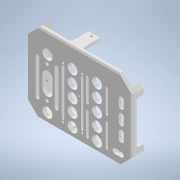
# Autodesk Inventor part: pcb_shell_1
Saved by Autodesk Inventor 2020 (Build 240168000, 168)
## iProperties
Created: 2019-07-14
Part Number: pcb_shell_1
Material: Generic
Document SubType Name: Modeling
Designer: psrob
Density: 1 g/cm^3
Appearance: Default
Author: psrob
Autodesk Inventor part; units mm, degrees
(part 1 of 2)
ref_plane "YZ Plane" through (0, 0, 0) normal (1, 0, 0) x (0, 1, 0)
ref_plane "XZ Plane" through (0, 0, 0) normal (0, 1, 0) x (-1, 0, 0)
ref_plane "XY Plane" through (0, 0, 0) normal (0, 0, 1) x (1, 0, 0)
sketch "Sketch1" plane through (0, 0, 0) normal (0, 0, 1) x (1, 0, 0)
  circle A0 centre (-25.7325, -16.0275) radius 1.27 projected
  circle A1 centre (-25.7325, 9.3725) radius 1.27 projected
  circle A2 centre (-13.0275, 16.3575) radius 0.889 projected
  circle A3 centre (2.2125, 16.3575) radius 0.889 projected
  circle A4 centre (2.2125, -24.2825) radius 0.889 projected
  circle A5 centre (-13.0275, -24.2825) radius 0.889 projected
  circle A6 centre (28.3275, -23.6475) radius 0.65 projected
  circle A7 centre (33.3275, -23.6475) radius 0.65 projected
  circle A8 centre (33.3275, -13.4075) radius 0.65 projected
  circle A9 centre (33.3275, -8.4075) radius 0.65 projected
  circle A10 centre (33.3275, -1.9775) radius 0.65 projected
  circle A11 centre (33.3275, 3.0225) radius 0.65 projected
  circle A12 centre (33.3275, 9.4525) radius 0.65 projected
  circle A13 centre (33.3275, 14.4525) radius 0.65 projected
  circle A14 centre (-33.3425, 10.6425) radius 0.555 projected
  circle A15 centre (-33.3425, 8.1025) radius 0.555 projected
  circle A16 centre (-33.3425, 5.5625) radius 0.555 projected
  circle A17 centre (-33.3425, 3.0225) radius 0.555 projected
  circle A18 centre (-33.3425, 0.4825) radius 0.555 projected
  circle A19 centre (-33.3425, -2.0575) radius 0.555 projected
  circle A20 centre (-33.3425, -4.5975) radius 0.555 projected
  circle A21 centre (-33.3425, -7.1375) radius 0.555 projected
  circle A22 centre (-33.3425, -9.6775) radius 0.555 projected
  circle A23 centre (-33.3425, -12.2175) radius 0.555 projected
  circle A24 centre (-33.3425, -14.7575) radius 0.555 projected
  circle A25 centre (-33.3425, -17.2975) radius 0.555 projected
  circle A26 centre (-18.1125, -17.2975) radius 0.555 projected
  circle A27 centre (-18.1125, -14.7575) radius 0.555 projected
  circle A28 centre (-18.1125, -12.2175) radius 0.555 projected
  circle A29 centre (-18.1125, -9.6775) radius 0.555 projected
  circle A30 centre (-18.1125, -7.1375) radius 0.555 projected
  circle A31 centre (-18.1125, -4.5975) radius 0.555 projected
  circle A32 centre (-18.1125, -2.0575) radius 0.555 projected
  circle A33 centre (-18.1125, 0.4825) radius 0.555 projected
  circle A34 centre (-18.1125, 3.0225) radius 0.555 projected
  circle A35 centre (-18.1125, 5.5625) radius 0.555 projected
  circle A36 centre (-18.1125, 8.1025) radius 0.555 projected
  circle A37 centre (-18.1125, 10.6425) radius 0.555 projected
  circle A38 centre (2.2075, -21.7475) radius 0.4 projected
  circle A39 centre (2.2075, -19.1975) radius 0.4 projected
  circle A40 centre (2.2075, -16.6675) radius 0.4 projected
  circle A41 centre (2.2075, -14.1175) radius 0.4 projected
  circle A42 centre (2.2075, -11.5775) radius 0.4 projected
  circle A43 centre (2.2075, -9.0475) radius 0.4 projected
  circle A44 centre (2.2075, -6.4975) radius 0.4 projected
  circle A45 centre (2.2075, -3.9575) radius 0.4 projected
  circle A46 centre (2.2075, -1.4175) radius 0.4 projected
  circle A47 centre (2.2075, 1.1225) radius 0.4 projected
  circle A48 centre (2.2075, 3.6625) radius 0.4 projected
  circle A49 centre (2.2075, 6.2025) radius 0.4 projected
  circle A50 centre (2.2075, 8.7425) radius 0.4 projected
  circle A51 centre (2.2075, 11.2725) radius 0.4 projected
  circle A52 centre (2.2075, 13.8125) radius 0.4 projected
  circle A53 centre (-13.0225, 13.8125) radius 0.4 projected
  circle A54 centre (-13.0225, 11.2725) radius 0.4 projected
  circle A55 centre (-13.0225, 8.7425) radius 0.4 projected
  circle A56 centre (-13.0225, 6.2025) radius 0.4 projected
  circle A57 centre (-13.0225, 3.6625) radius 0.4 projected
  circle A58 centre (-13.0225, 1.1225) radius 0.4 projected
  circle A59 centre (-13.0225, -1.4175) radius 0.4 projected
  circle A60 centre (-13.0225, -3.9575) radius 0.4 projected
  circle A61 centre (-13.0225, -6.4975) radius 0.4 projected
  circle A62 centre (-13.0225, -9.0475) radius 0.4 projected
  circle A63 centre (-13.0225, -11.5775) radius 0.4 projected
  circle A64 centre (-13.0225, -14.1175) radius 0.4 projected
  circle A65 centre (-13.0225, -16.6675) radius 0.4 projected
  circle A66 centre (-13.0225, -19.1975) radius 0.4 projected
  circle A67 centre (-13.0225, -21.7475) radius 0.4 projected
  circle A68 centre (21.8975, -7.1375) radius 0.35 projected
  circle A69 centre (21.8975, 16.3625) radius 0.35 projected
  circle A70 centre (21.8975, -9.6775) radius 0.3 projected
  circle A71 centre (6.4075, -14.7575) radius 0.3 projected
  circle A72 centre (6.4075, -22.3775) radius 0.3 projected
  circle A73 centre (6.4075, -7.1375) radius 0.3 projected
  circle A74 centre (6.4075, -24.9175) radius 0.3 projected
  circle A75 centre (21.8975, -24.9175) radius 0.3 projected
  circle A76 centre (21.8975, -12.2175) radius 0.3 projected
  circle A77 centre (6.4075, -19.8375) radius 0.3 projected
  circle A78 centre (6.4075, -17.2975) radius 0.3 projected
  circle A79 centre (21.8975, -19.8375) radius 0.3 projected
  circle A80 centre (21.8975, -22.3775) radius 0.3 projected
  circle A81 centre (6.4075, -9.6775) radius 0.3 projected
  circle A82 centre (6.4075, -12.2175) radius 0.3 projected
  circle A83 centre (21.8975, -17.2975) radius 0.3 projected
  circle A84 centre (21.8975, -14.7575) radius 0.3 projected
  circle A85 centre (21.8975, 13.8125) radius 0.3 projected
  circle A86 centre (6.4075, 8.7425) radius 0.3 projected
  circle A87 centre (6.4075, 1.1225) radius 0.3 projected
  circle A88 centre (6.4075, 16.3625) radius 0.3 projected
  circle A89 centre (6.4075, -1.4175) radius 0.3 projected
  circle A90 centre (21.8975, -1.4175) radius 0.3 projected
  circle A91 centre (21.8975, 11.2725) radius 0.3 projected
  circle A92 centre (6.4075, 3.6625) radius 0.3 projected
  circle A93 centre (6.4075, 6.2025) radius 0.3 projected
  circle A94 centre (21.8975, 3.6625) radius 0.3 projected
  circle A95 centre (21.8975, 1.1225) radius 0.3 projected
  circle A96 centre (6.4075, 13.8125) radius 0.3 projected
  circle A97 centre (6.4075, 11.2725) radius 0.3 projected
  circle A98 centre (21.8975, 6.2025) radius 0.3 projected
  circle A99 centre (21.8975, 8.7425) radius 0.3 projected
  circle A100 centre (11.0517, 18.7705) radius 0.175 projected
  circle A101 centre (4.7779, 21.7423) radius 0.175 projected
  circle A102 centre (15.3443, 11.8363) radius 0.175 projected
  circle A103 centre (29.2127, 21.7423) radius 0.175 projected
  circle A104 centre (-2.8167, 21.4121) radius 0.175 projected
  circle A105 centre (-15.0341, 10.8457) radius 0.175 projected
  line L0 (37.1375, -27.4575) -> (-37.1375, -27.4575) projected
  line L1 (37.1375, 27.4575) -> (37.1375, -27.4575) projected
  line L2 (-37.1375, 27.4575) -> (37.1375, 27.4575) projected
  line L3 (-37.1375, -27.4575) -> (-37.1375, 27.4575) projected
  line L4 (-39, 29) -> (39, 29)
  line L5 (39, 29) -> (39, -29)
  line L6 (39, -29) -> (-39, -29)
  line L7 (-39, -29) -> (-39, 29)
  line L8 (-39, 29) -> (39, -29) construction
  line L9 (39, 29) -> (-39, -29) construction
  line L10 (-42, 31.5) -> (42, 31.5)
  line L11 (42, 31.5) -> (42, -31.5)
  line L12 (42, -31.5) -> (-42, -31.5)
  line L13 (-42, -31.5) -> (-42, 31.5)
  line L14 (-42, 31.5) -> (42, -31.5) construction
  line L15 (42, 31.5) -> (-42, -31.5) construction
  point P0 (0, 0)
  dimension "d0" = 78
  dimension "d1" = 58
  dimension "d2" = 84
  dimension "d3" = 63
  constraints: 24 end point, 4 midpoint, 4 parallel, 3 perpendicular, 1 horizontal
  measures "d0" distance of L4.start L4.end
  measures "d1" distance of L4.end L5.end
  measures "d2" distance of L10.start L10.end
  measures "d3" distance of L10.end L11.end
extrude "Extrusion1" add sketch "Sketch1" along normal blind 3 contours A0 | A1 | A2 | A3 | A4 | A5 | A6 | A7 | A8 | A9 | A10 | A11 | A12 | A13 | A14 | A15 | A16 | A17 | A18 | A19 | A20 | A21 | A22 | A23 | A24 | A25 | A26 | A27 | A28 | A29 | A30 | A31 | A32 | A33 | A34 | A35 | A36 | A37 | A38 | A39 | A40 | A41 | A42 | A43 | A44 | A45 | A46 | A47 | A48 | A49 | A50 | A51 | A52 | A53 | A54 | A55 | A56 | A57 | A58 | A59 | A60 | A61 | A62 | A63 | A64 | A65 | A66 | A67 | A68 | A69 | A70 | A71 | A72 | A73 | A74 | A75 | A76 | A77 | A78 | A79 | A80 | A81 | A82 | A83 | A84 | A85 | A86 | A87 | A88 | A89 | A90 | A91 | A92 | A93 | A94 | A95 | A96 | A97 | A98 | A99 | A100 | A101 | A102 | A103 | A104 | A105 | L0 L3 L2 L1 | L4 L5 L6 L7 | L10 L11 L12 L13
sketch "Sketch2" plane through (0, 0, 0) normal (0, 0, -1) x (-1, 0, 0)
  line L0 (42, -31.5) -> (-42, -31.5) projected
  line L1 (42, 31.5) -> (42, -31.5) projected
  line L2 (-42, 31.5) -> (42, 31.5) projected
  line L3 (-42, -31.5) -> (-42, 31.5) projected
  line L4 (39, -29) -> (-39, -29)
  line L5 (-39, -29) -> (-39, 29)
  line L6 (-39, 29) -> (39, 29)
  line L7 (39, 29) -> (39, -29)
  line L8 (39, -29) -> (-39, 29) construction
  line L9 (-39, -29) -> (39, 29) construction
  point P0 (0, 0)
  dimension "d6" = 78
  dimension "d7" = 58
  constraints: 12 end point, 2 midpoint, 2 parallel, 1 horizontal, 1 perpendicular
  measures "d6" distance of L4.start L4.end
  measures "d7" distance of L4.end L5.end
extrude "Extrusion2" add sketch "Sketch2" along normal blind 14
sketch "Sketch3" plane through (0, 0, 3) normal (0, 0, 1) x (1, 0, 0)
  circle A0 centre (-25.7325, -16.0275) radius 1.27 projected
  circle A1 centre (-25.7325, 9.3725) radius 1.27 projected
  circle A2 centre (-13.0275, 16.3575) radius 0.889 projected
  circle A3 centre (2.2125, 16.3575) radius 0.889 projected
  circle A4 centre (2.2125, -24.2825) radius 0.889 projected
  circle A5 centre (-13.0275, -24.2825) radius 0.889 projected
  circle A6 centre (28.3275, -23.6475) radius 0.65 projected
  circle A7 centre (33.3275, -23.6475) radius 0.65 projected
  circle A8 centre (33.3275, -13.4075) radius 0.65 projected
  circle A9 centre (33.3275, -8.4075) radius 0.65 projected
  circle A10 centre (33.3275, -1.9775) radius 0.65 projected
  circle A11 centre (33.3275, 3.0225) radius 0.65 projected
  circle A12 centre (33.3275, 9.4525) radius 0.65 projected
  circle A13 centre (33.3275, 14.4525) radius 0.65 projected
  circle A14 centre (-33.3425, 10.6425) radius 0.555 projected
  circle A15 centre (-33.3425, 8.1025) radius 0.555 projected
  circle A16 centre (-33.3425, 5.5625) radius 0.555 projected
  circle A17 centre (-33.3425, 3.0225) radius 0.555 projected
  circle A18 centre (-33.3425, 0.4825) radius 0.555 projected
  circle A19 centre (-33.3425, -2.0575) radius 0.555 projected
  circle A20 centre (-33.3425, -4.5975) radius 0.555 projected
  circle A21 centre (-33.3425, -7.1375) radius 0.555 projected
  circle A22 centre (-33.3425, -9.6775) radius 0.555 projected
  circle A23 centre (-33.3425, -12.2175) radius 0.555 projected
  circle A24 centre (-33.3425, -14.7575) radius 0.555 projected
  circle A25 centre (-33.3425, -17.2975) radius 0.555 projected
  circle A26 centre (-18.1125, -17.2975) radius 0.555 projected
  circle A27 centre (-18.1125, -14.7575) radius 0.555 projected
  circle A28 centre (-18.1125, -12.2175) radius 0.555 projected
  circle A29 centre (-18.1125, -9.6775) radius 0.555 projected
  circle A30 centre (-18.1125, -7.1375) radius 0.555 projected
  circle A31 centre (-18.1125, -4.5975) radius 0.555 projected
  circle A32 centre (-18.1125, -2.0575) radius 0.555 projected
  circle A33 centre (-18.1125, 0.4825) radius 0.555 projected
  circle A34 centre (-18.1125, 3.0225) radius 0.555 projected
  circle A35 centre (-18.1125, 5.5625) radius 0.555 projected
  circle A36 centre (-18.1125, 8.1025) radius 0.555 projected
  circle A37 centre (-18.1125, 10.6425) radius 0.555 projected
  circle A38 centre (2.2075, -21.7475) radius 0.4 projected
  circle A39 centre (2.2075, -19.1975) radius 0.4 projected
  circle A40 centre (2.2075, -16.6675) radius 0.4 projected
  circle A41 centre (2.2075, -14.1175) radius 0.4 projected
  circle A42 centre (2.2075, -11.5775) radius 0.4 projected
  circle A43 centre (2.2075, -9.0475) radius 0.4 projected
  circle A44 centre (2.2075, -6.4975) radius 0.4 projected
  circle A45 centre (2.2075, -3.9575) radius 0.4 projected
  circle A46 centre (2.2075, -1.4175) radius 0.4 projected
  circle A47 centre (2.2075, 1.1225) radius 0.4 projected
  circle A48 centre (2.2075, 3.6625) radius 0.4 projected
  circle A49 centre (2.2075, 6.2025) radius 0.4 projected
  circle A50 centre (2.2075, 8.7425) radius 0.4 projected
  circle A51 centre (2.2075, 11.2725) radius 0.4 projected
  circle A52 centre (2.2075, 13.8125) radius 0.4 projected
  circle A53 centre (-13.0225, 13.8125) radius 0.4 projected
  circle A54 centre (-13.0225, 11.2725) radius 0.4 projected
  circle A55 centre (-13.0225, 8.7425) radius 0.4 projected
  circle A56 centre (-13.0225, 6.2025) radius 0.4 projected
  circle A57 centre (-13.0225, 3.6625) radius 0.4 projected
  circle A58 centre (-13.0225, 1.1225) radius 0.4 projected
  circle A59 centre (-13.0225, -1.4175) radius 0.4 projected
  circle A60 centre (-13.0225, -3.9575) radius 0.4 projected
  circle A61 centre (-13.0225, -6.4975) radius 0.4 projected
  circle A62 centre (-13.0225, -9.0475) radius 0.4 projected
  circle A63 centre (-13.0225, -11.5775) radius 0.4 projected
  circle A64 centre (-13.0225, -14.1175) radius 0.4 projected
  circle A65 centre (-13.0225, -16.6675) radius 0.4 projected
  circle A66 centre (-13.0225, -19.1975) radius 0.4 projected
  circle A67 centre (-13.0225, -21.7475) radius 0.4 projected
  circle A68 centre (21.8975, -7.1375) radius 0.35 projected
  circle A69 centre (21.8975, 16.3625) radius 0.35 projected
  circle A70 centre (21.8975, -9.6775) radius 0.3 projected
  circle A71 centre (6.4075, -14.7575) radius 0.3 projected
  circle A72 centre (6.4075, -22.3775) radius 0.3 projected
  circle A73 centre (6.4075, -7.1375) radius 0.3 projected
  circle A74 centre (6.4075, -24.9175) radius 0.3 projected
  circle A75 centre (21.8975, -24.9175) radius 0.3 projected
  circle A76 centre (21.8975, -12.2175) radius 0.3 projected
  circle A77 centre (6.4075, -19.8375) radius 0.3 projected
  circle A78 centre (6.4075, -17.2975) radius 0.3 projected
  circle A79 centre (21.8975, -19.8375) radius 0.3 projected
  circle A80 centre (21.8975, -22.3775) radius 0.3 projected
  circle A81 centre (6.4075, -9.6775) radius 0.3 projected
  circle A82 centre (6.4075, -12.2175) radius 0.3 projected
  circle A83 centre (21.8975, -17.2975) radius 0.3 projected
  circle A84 centre (21.8975, -14.7575) radius 0.3 projected
  circle A85 centre (21.8975, 13.8125) radius 0.3 projected
  circle A86 centre (6.4075, 8.7425) radius 0.3 projected
  circle A87 centre (6.4075, 1.1225) radius 0.3 projected
  circle A88 centre (6.4075, 16.3625) radius 0.3 projected
  circle A89 centre (6.4075, -1.4175) radius 0.3 projected
  circle A90 centre (21.8975, -1.4175) radius 0.3 projected
  circle A91 centre (21.8975, 11.2725) radius 0.3 projected
  circle A92 centre (6.4075, 3.6625) radius 0.3 projected
  circle A93 centre (6.4075, 6.2025) radius 0.3 projected
  circle A94 centre (21.8975, 3.6625) radius 0.3 projected
  circle A95 centre (21.8975, 1.1225) radius 0.3 projected
  circle A96 centre (6.4075, 13.8125) radius 0.3 projected
  circle A97 centre (6.4075, 11.2725) radius 0.3 projected
  circle A98 centre (21.8975, 6.2025) radius 0.3 projected
  circle A99 centre (21.8975, 8.7425) radius 0.3 projected
  circle A100 centre (11.0517, 18.7705) radius 0.175 projected
  circle A101 centre (4.7779, 21.7423) radius 0.175 projected
  circle A102 centre (15.3443, 11.8363) radius 0.175 projected
  circle A103 centre (29.2127, 21.7423) radius 0.175 projected
  circle A104 centre (-2.8167, 21.4121) radius 0.175 projected
  circle A105 centre (-15.0341, 10.8457) radius 0.175 projected
  line L0 (37.1375, -27.4575) -> (-37.1375, -27.4575) projected
  line L1 (-37.1375, -27.4575) -> (-37.1375, 27.4575) projected
  line L2 (-37.1375, 27.4575) -> (37.1375, 27.4575) projected
  line L3 (37.1375, 27.4575) -> (37.1375, -27.4575) projected
  point P0 (0, 0)
extrude "Extrusion3" cut sketch "Sketch3" against normal blind 14 contours A2 | A3 | A4 | A5
sketch "Sketch4" plane through (0, 0, 3) normal (0, 0, 1) x (1, 0, 0)
  circle A0 centre (-25.7325, -16.0275) radius 1.27 projected
  circle A1 centre (-25.7325, 9.3725) radius 1.27 projected
  circle A2 centre (-13.0275, 16.3575) radius 0.889 projected
  circle A3 centre (2.2125, 16.3575) radius 0.889 projected
  circle A4 centre (2.2125, -24.2825) radius 0.889 projected
  circle A5 centre (-13.0275, -24.2825) radius 0.889 projected
  circle A6 centre (28.3275, -23.6475) radius 0.65 projected
  circle A7 centre (33.3275, -23.6475) radius 0.65 projected
  circle A8 centre (33.3275, -13.4075) radius 0.65 projected
  circle A9 centre (33.3275, -8.4075) radius 0.65 projected
  circle A10 centre (33.3275, -1.9775) radius 0.65 projected
  circle A11 centre (33.3275, 3.0225) radius 0.65 projected
  circle A12 centre (33.3275, 9.4525) radius 0.65 projected
  circle A13 centre (33.3275, 14.4525) radius 0.65 projected
  circle A14 centre (-33.3425, 10.6425) radius 0.555 projected
  circle A15 centre (-33.3425, 8.1025) radius 0.555 projected
  circle A16 centre (-33.3425, 5.5625) radius 0.555 projected
  circle A17 centre (-33.3425, 3.0225) radius 0.555 projected
  circle A18 centre (-33.3425, 0.4825) radius 0.555 projected
  circle A19 centre (-33.3425, -2.0575) radius 0.555 projected
  circle A20 centre (-33.3425, -4.5975) radius 0.555 projected
  circle A21 centre (-33.3425, -7.1375) radius 0.555 projected
  circle A22 centre (-33.3425, -9.6775) radius 0.555 projected
  circle A23 centre (-33.3425, -12.2175) radius 0.555 projected
  circle A24 centre (-33.3425, -14.7575) radius 0.555 projected
  circle A25 centre (-33.3425, -17.2975) radius 0.555 projected
  circle A26 centre (-18.1125, -17.2975) radius 0.555 projected
  circle A27 centre (-18.1125, -14.7575) radius 0.555 projected
  circle A28 centre (-18.1125, -12.2175) radius 0.555 projected
  circle A29 centre (-18.1125, -9.6775) radius 0.555 projected
  circle A30 centre (-18.1125, -7.1375) radius 0.555 projected
  circle A31 centre (-18.1125, -4.5975) radius 0.555 projected
  circle A32 centre (-18.1125, -2.0575) radius 0.555 projected
  circle A33 centre (-18.1125, 0.4825) radius 0.555 projected
  circle A34 centre (-18.1125, 3.0225) radius 0.555 projected
  circle A35 centre (-18.1125, 5.5625) radius 0.555 projected
  circle A36 centre (-18.1125, 8.1025) radius 0.555 projected
  circle A37 centre (-18.1125, 10.6425) radius 0.555 projected
  circle A38 centre (2.2075, -21.7475) radius 0.4 projected
  circle A39 centre (2.2075, -19.1975) radius 0.4 projected
  circle A40 centre (2.2075, -16.6675) radius 0.4 projected
  circle A41 centre (2.2075, -14.1175) radius 0.4 projected
  circle A42 centre (2.2075, -11.5775) radius 0.4 projected
  circle A43 centre (2.2075, -9.0475) radius 0.4 projected
  circle A44 centre (2.2075, -6.4975) radius 0.4 projected
  circle A45 centre (2.2075, -3.9575) radius 0.4 projected
  circle A46 centre (2.2075, -1.4175) radius 0.4 projected
  circle A47 centre (2.2075, 1.1225) radius 0.4 projected
  circle A48 centre (2.2075, 3.6625) radius 0.4 projected
  circle A49 centre (2.2075, 6.2025) radius 0.4 projected
  circle A50 centre (2.2075, 8.7425) radius 0.4 projected
  circle A51 centre (2.2075, 11.2725) radius 0.4 projected
  circle A52 centre (2.2075, 13.8125) radius 0.4 projected
  circle A53 centre (-13.0225, 13.8125) radius 0.4 projected
  circle A54 centre (-13.0225, 11.2725) radius 0.4 projected
  circle A55 centre (-13.0225, 8.7425) radius 0.4 projected
  circle A56 centre (-13.0225, 6.2025) radius 0.4 projected
  circle A57 centre (-13.0225, 3.6625) radius 0.4 projected
  circle A58 centre (-13.0225, 1.1225) radius 0.4 projected
  circle A59 centre (-13.0225, -1.4175) radius 0.4 projected
  circle A60 centre (-13.0225, -3.9575) radius 0.4 projected
  circle A61 centre (-13.0225, -6.4975) radius 0.4 projected
  circle A62 centre (-13.0225, -9.0475) radius 0.4 projected
  circle A63 centre (-13.0225, -11.5775) radius 0.4 projected
  circle A64 centre (-13.0225, -14.1175) radius 0.4 projected
  circle A65 centre (-13.0225, -16.6675) radius 0.4 projected
  circle A66 centre (-13.0225, -19.1975) radius 0.4 projected
  circle A67 centre (-13.0225, -21.7475) radius 0.4 projected
  circle A68 centre (21.8975, -7.1375) radius 0.35 projected
  circle A69 centre (21.8975, 16.3625) radius 0.35 projected
  circle A70 centre (21.8975, -9.6775) radius 0.3 projected
  circle A71 centre (6.4075, -14.7575) radius 0.3 projected
  circle A72 centre (6.4075, -22.3775) radius 0.3 projected
  circle A73 centre (6.4075, -7.1375) radius 0.3 projected
  circle A74 centre (6.4075, -24.9175) radius 0.3 projected
  circle A75 centre (21.8975, -24.9175) radius 0.3 projected
  circle A76 centre (21.8975, -12.2175) radius 0.3 projected
  circle A77 centre (6.4075, -19.8375) radius 0.3 projected
  circle A78 centre (6.4075, -17.2975) radius 0.3 projected
  circle A79 centre (21.8975, -19.8375) radius 0.3 projected
  circle A80 centre (21.8975, -22.3775) radius 0.3 projected
  circle A81 centre (6.4075, -9.6775) radius 0.3 projected
  circle A82 centre (6.4075, -12.2175) radius 0.3 projected
  circle A83 centre (21.8975, -17.2975) radius 0.3 projected
  circle A84 centre (21.8975, -14.7575) radius 0.3 projected
  circle A85 centre (21.8975, 13.8125) radius 0.3 projected
  circle A86 centre (6.4075, 8.7425) radius 0.3 projected
  circle A87 centre (6.4075, 1.1225) radius 0.3 projected
  circle A88 centre (6.4075, 16.3625) radius 0.3 projected
  circle A89 centre (6.4075, -1.4175) radius 0.3 projected
  circle A90 centre (21.8975, -1.4175) radius 0.3 projected
  circle A91 centre (21.8975, 11.2725) radius 0.3 projected
  circle A92 centre (6.4075, 3.6625) radius 0.3 projected
  circle A93 centre (6.4075, 6.2025) radius 0.3 projected
  circle A94 centre (21.8975, 3.6625) radius 0.3 projected
  circle A95 centre (21.8975, 1.1225) radius 0.3 projected
  circle A96 centre (6.4075, 13.8125) radius 0.3 projected
  circle A97 centre (6.4075, 11.2725) radius 0.3 projected
  circle A98 centre (21.8975, 6.2025) radius 0.3 projected
  circle A99 centre (21.8975, 8.7425) radius 0.3 projected
  circle A100 centre (11.0517, 18.7705) radius 0.175 projected
  circle A101 centre (4.7779, 21.7423) radius 0.175 projected
  circle A102 centre (15.3443, 11.8363) radius 0.175 projected
  circle A103 centre (29.2127, 21.7423) radius 0.175 projected
  circle A104 centre (-2.8167, 21.4121) radius 0.175 projected
  circle A105 centre (-15.0341, 10.8457) radius 0.175 projected
  line L0 (37.1375, -27.4575) -> (-37.1375, -27.4575) projected
  line L1 (-37.1375, -27.4575) -> (-37.1375, 27.4575) projected
  line L2 (-37.1375, 27.4575) -> (37.1375, 27.4575) projected
  line L3 (37.1375, 27.4575) -> (37.1375, -27.4575) projected
  point P0 (0, 0)
extrude "Extrusion4" cut sketch "Sketch4" against normal blind 14 contours A0 | A1
sketch "Sketch5" plane through (0, 0, 3) normal (0, 0, 1) x (1, 0, 0)
  circle A0 centre (-25.7325, -16.0275) radius 1.27 projected
  circle A1 centre (-25.7325, 9.3725) radius 1.27 projected
  circle A2 centre (-13.0275, 16.3575) radius 0.889 projected
  circle A3 centre (2.2125, 16.3575) radius 0.889 projected
  circle A4 centre (2.2125, -24.2825) radius 0.889 projected
  circle A5 centre (-13.0275, -24.2825) radius 0.889 projected
  circle A6 centre (28.3275, -23.6475) radius 0.65 projected
  circle A7 centre (33.3275, -23.6475) radius 0.65 projected
  circle A8 centre (33.3275, -13.4075) radius 0.65 projected
  circle A9 centre (33.3275, -8.4075) radius 0.65 projected
  circle A10 centre (33.3275, -1.9775) radius 0.65 projected
  circle A11 centre (33.3275, 3.0225) radius 0.65 projected
  circle A12 centre (33.3275, 9.4525) radius 0.65 projected
  circle A13 centre (33.3275, 14.4525) radius 0.65 projected
  circle A14 centre (-33.3425, 10.6425) radius 0.555 projected
  circle A15 centre (-33.3425, 8.1025) radius 0.555 projected
  circle A16 centre (-33.3425, 5.5625) radius 0.555 projected
  circle A17 centre (-33.3425, 3.0225) radius 0.555 projected
  circle A18 centre (-33.3425, 0.4825) radius 0.555 projected
  circle A19 centre (-33.3425, -2.0575) radius 0.555 projected
  circle A20 centre (-33.3425, -4.5975) radius 0.555 projected
  circle A21 centre (-33.3425, -7.1375) radius 0.555 projected
  circle A22 centre (-33.3425, -9.6775) radius 0.555 projected
  circle A23 centre (-33.3425, -12.2175) radius 0.555 projected
  circle A24 centre (-33.3425, -14.7575) radius 0.555 projected
  circle A25 centre (-33.3425, -17.2975) radius 0.555 projected
  circle A26 centre (-18.1125, -17.2975) radius 0.555 projected
  circle A27 centre (-18.1125, -14.7575) radius 0.555 projected
  circle A28 centre (-18.1125, -12.2175) radius 0.555 projected
  circle A29 centre (-18.1125, -9.6775) radius 0.555 projected
  circle A30 centre (-18.1125, -7.1375) radius 0.555 projected
  circle A31 centre (-18.1125, -4.5975) radius 0.555 projected
  circle A32 centre (-18.1125, -2.0575) radius 0.555 projected
  circle A33 centre (-18.1125, 0.4825) radius 0.555 projected
  circle A34 centre (-18.1125, 3.0225) radius 0.555 projected
  circle A35 centre (-18.1125, 5.5625) radius 0.555 projected
  circle A36 centre (-18.1125, 8.1025) radius 0.555 projected
  circle A37 centre (-18.1125, 10.6425) radius 0.555 projected
  circle A38 centre (2.2075, -21.7475) radius 0.4 projected
  circle A39 centre (2.2075, -19.1975) radius 0.4 projected
  circle A40 centre (2.2075, -16.6675) radius 0.4 projected
  circle A41 centre (2.2075, -14.1175) radius 0.4 projected
  circle A42 centre (2.2075, -11.5775) radius 0.4 projected
  circle A43 centre (2.2075, -9.0475) radius 0.4 projected
  circle A44 centre (2.2075, -6.4975) radius 0.4 projected
  circle A45 centre (2.2075, -3.9575) radius 0.4 projected
  circle A46 centre (2.2075, -1.4175) radius 0.4 projected
  circle A47 centre (2.2075, 1.1225) radius 0.4 projected
  circle A48 centre (2.2075, 3.6625) radius 0.4 projected
  circle A49 centre (2.2075, 6.2025) radius 0.4 projected
  circle A50 centre (2.2075, 8.7425) radius 0.4 projected
  circle A51 centre (2.2075, 11.2725) radius 0.4 projected
  circle A52 centre (2.2075, 13.8125) radius 0.4 projected
  circle A53 centre (-13.0225, 13.8125) radius 0.4 projected
  circle A54 centre (-13.0225, 11.2725) radius 0.4 projected
  circle A55 centre (-13.0225, 8.7425) radius 0.4 projected
  circle A56 centre (-13.0225, 6.2025) radius 0.4 projected
  circle A57 centre (-13.0225, 3.6625) radius 0.4 projected
  circle A58 centre (-13.0225, 1.1225) radius 0.4 projected
  circle A59 centre (-13.0225, -1.4175) radius 0.4 projected
  circle A60 centre (-13.0225, -3.9575) radius 0.4 projected
  circle A61 centre (-13.0225, -6.4975) radius 0.4 projected
  circle A62 centre (-13.0225, -9.0475) radius 0.4 projected
  circle A63 centre (-13.0225, -11.5775) radius 0.4 projected
  circle A64 centre (-13.0225, -14.1175) radius 0.4 projected
  circle A65 centre (-13.0225, -16.6675) radius 0.4 projected
  circle A66 centre (-13.0225, -19.1975) radius 0.4 projected
  circle A67 centre (-13.0225, -21.7475) radius 0.4 projected
  circle A68 centre (21.8975, -7.1375) radius 0.35 projected
  circle A69 centre (21.8975, 16.3625) radius 0.35 projected
  circle A70 centre (21.8975, -9.6775) radius 0.3 projected
  circle A71 centre (6.4075, -14.7575) radius 0.3 projected
  circle A72 centre (6.4075, -22.3775) radius 0.3 projected
  circle A73 centre (6.4075, -7.1375) radius 0.3 projected
  circle A74 centre (6.4075, -24.9175) radius 0.3 projected
  circle A75 centre (21.8975, -24.9175) radius 0.3 projected
  circle A76 centre (21.8975, -12.2175) radius 0.3 projected
  circle A77 centre (6.4075, -19.8375) radius 0.3 projected
  circle A78 centre (6.4075, -17.2975) radius 0.3 projected
  circle A79 centre (21.8975, -19.8375) radius 0.3 projected
  circle A80 centre (21.8975, -22.3775) radius 0.3 projected
  circle A81 centre (6.4075, -9.6775) radius 0.3 projected
  circle A82 centre (6.4075, -12.2175) radius 0.3 projected
  circle A83 centre (21.8975, -17.2975) radius 0.3 projected
  circle A84 centre (21.8975, -14.7575) radius 0.3 projected
  circle A85 centre (21.8975, 13.8125) radius 0.3 projected
  circle A86 centre (6.4075, 8.7425) radius 0.3 projected
  circle A87 centre (6.4075, 1.1225) radius 0.3 projected
  circle A88 centre (6.4075, 16.3625) radius 0.3 projected
  circle A89 centre (6.4075, -1.4175) radius 0.3 projected
  circle A90 centre (21.8975, -1.4175) radius 0.3 projected
  circle A91 centre (21.8975, 11.2725) radius 0.3 projected
  circle A92 centre (6.4075, 3.6625) radius 0.3 projected
  circle A93 centre (6.4075, 6.2025) radius 0.3 projected
  circle A94 centre (21.8975, 3.6625) radius 0.3 projected
  circle A95 centre (21.8975, 1.1225) radius 0.3 projected
  circle A96 centre (6.4075, 13.8125) radius 0.3 projected
  circle A97 centre (6.4075, 11.2725) radius 0.3 projected
  circle A98 centre (21.8975, 6.2025) radius 0.3 projected
  circle A99 centre (21.8975, 8.7425) radius 0.3 projected
  circle A100 centre (11.0517, 18.7705) radius 0.175 projected
  circle A101 centre (4.7779, 21.7423) radius 0.175 projected
  circle A102 centre (15.3443, 11.8363) radius 0.175 projected
  circle A103 centre (29.2127, 21.7423) radius 0.175 projected
  circle A104 centre (-2.8167, 21.4121) radius 0.175 projected
  circle A105 centre (-15.0341, 10.8457) radius 0.175 projected
  line L0 (37.1375, -27.4575) -> (-37.1375, -27.4575) projected
  line L1 (-37.1375, -27.4575) -> (-37.1375, 27.4575) projected
  line L2 (-37.1375, 27.4575) -> (37.1375, 27.4575) projected
  line L3 (37.1375, 27.4575) -> (37.1375, -27.4575) projected
  line L4 (-33.3425, 10.6425) -> (-33.3425, -17.2975) construction
  line L5 (-34.8425, 10.6425) -> (-34.8425, -17.2975)
  line L6 (-31.8425, -17.2975) -> (-31.8425, 10.6425)
  arc A106 (-31.8425, 10.6425) -> (-34.8425, 10.6425) centre (-33.3425, 10.6425) ccw
  arc A107 (-34.8425, -17.2975) -> (-31.8425, -17.2975) centre (-33.3425, -17.2975) ccw
  line L7 (-18.1125, 10.6425) -> (-18.1125, -17.2975) construction
  line L8 (-19.6125, 10.6425) -> (-19.6125, -17.2975)
  line L9 (-16.6125, -17.2975) -> (-16.6125, 10.6425)
  arc A108 (-16.6125, 10.6425) -> (-19.6125, 10.6425) centre (-18.1125, 10.6425) ccw
  arc A109 (-19.6125, -17.2975) -> (-16.6125, -17.2975) centre (-18.1125, -17.2975) ccw
  line L10 (-13.0225, 13.8125) -> (-13.0225, -21.7475) construction
  line L11 (-14.0225, 13.8125) -> (-14.0225, -21.7475)
  line L12 (-12.0225, -21.7475) -> (-12.0225, 13.8125)
  arc A110 (-12.0225, 13.8125) -> (-14.0225, 13.8125) centre (-13.0225, 13.8125) ccw
  arc A111 (-14.0225, -21.7475) -> (-12.0225, -21.7475) centre (-13.0225, -21.7475) ccw
  line L13 (2.2075, 13.8125) -> (2.2075, -21.7475) construction
  line L14 (1.2075, 13.8125) -> (1.2075, -21.7475)
  line L15 (3.2075, -21.7475) -> (3.2075, 13.8125)
  arc A112 (3.2075, 13.8125) -> (1.2075, 13.8125) centre (2.2075, 13.8125) ccw
  arc A113 (1.2075, -21.7475) -> (3.2075, -21.7475) centre (2.2075, -21.7475) ccw
  line L16 (6.4075, 16.3625) -> (6.4075, -1.4175) construction
  line L17 (5.4075, 16.3625) -> (5.4075, -1.4175)
  line L18 (7.4075, -1.4175) -> (7.4075, 16.3625)
  arc A114 (7.4075, 16.3625) -> (5.4075, 16.3625) centre (6.4075, 16.3625) ccw
  arc A115 (5.4075, -1.4175) -> (7.4075, -1.4175) centre (6.4075, -1.4175) ccw
  line L19 (21.8975, 16.3625) -> (21.8975, -1.4175) construction
  line L20 (20.8975, 16.3625) -> (20.8975, -1.4175)
  line L21 (22.8975, -1.4175) -> (22.8975, 16.3625)
  arc A116 (22.8975, 16.3625) -> (20.8975, 16.3625) centre (21.8975, 16.3625) ccw
  arc A117 (20.8975, -1.4175) -> (22.8975, -1.4175) centre (21.8975, -1.4175) ccw
  line L22 (6.4075, -7.1375) -> (6.4075, -24.9175) construction
  line L23 (5.4075, -7.1375) -> (5.4075, -24.9175)
  line L24 (7.4075, -24.9175) -> (7.4075, -7.1375)
  arc A118 (7.4075, -7.1375) -> (5.4075, -7.1375) centre (6.4075, -7.1375) ccw
  arc A119 (5.4075, -24.9175) -> (7.4075, -24.9175) centre (6.4075, -24.9175) ccw
  line L25 (21.8975, -7.1375) -> (21.8975, -24.9175) construction
  line L26 (20.8975, -7.1375) -> (20.8975, -24.9175)
  line L27 (22.8975, -24.9175) -> (22.8975, -7.1375)
  arc A120 (22.8975, -7.1375) -> (20.8975, -7.1375) centre (21.8975, -7.1375) ccw
  arc A121 (20.8975, -24.9175) -> (22.8975, -24.9175) centre (21.8975, -24.9175) ccw
  line L28 (33.3275, 14.4525) -> (33.3275, 9.4525) construction
  line L29 (31.3275, 14.4525) -> (31.3275, 9.4525)
  line L30 (35.3275, 9.4525) -> (35.3275, 14.4525)
  arc A122 (35.3275, 14.4525) -> (31.3275, 14.4525) centre (33.3275, 14.4525) ccw
  arc A123 (31.3275, 9.4525) -> (35.3275, 9.4525) centre (33.3275, 9.4525) ccw
  line L31 (33.3275, 3.0225) -> (33.3275, -1.9775) construction
  line L32 (31.3275, 3.0225) -> (31.3275, -1.9775)
  line L33 (35.3275, -1.9775) -> (35.3275, 3.0225)
  arc A124 (35.3275, 3.0225) -> (31.3275, 3.0225) centre (33.3275, 3.0225) ccw
  arc A125 (31.3275, -1.9775) -> (35.3275, -1.9775) centre (33.3275, -1.9775) ccw
  line L34 (33.3275, -8.4075) -> (33.3275, -13.4075) construction
  line L35 (31.3275, -8.4075) -> (31.3275, -13.4075)
  line L36 (35.3275, -13.4075) -> (35.3275, -8.4075)
  arc A126 (35.3275, -8.4075) -> (31.3275, -8.4075) centre (33.3275, -8.4075) ccw
  arc A127 (31.3275, -13.4075) -> (35.3275, -13.4075) centre (33.3275, -13.4075) ccw
  line L37 (28.3275, -23.6475) -> (33.3275, -23.6475) construction
  line L38 (28.3275, -25.6475) -> (33.3275, -25.6475)
  line L39 (33.3275, -21.6475) -> (28.3275, -21.6475)
  arc A128 (28.3275, -21.6475) -> (28.3275, -25.6475) centre (28.3275, -23.6475) ccw
  arc A129 (33.3275, -25.6475) -> (33.3275, -21.6475) centre (33.3275, -23.6475) ccw
  point P0 (0, 0)
  point P1 (-33.3425, -3.3275)
  point P2 (-18.1125, -3.3275)
  point P3 (-13.0225, -3.9675)
  point P4 (2.2075, -3.9675)
  point P5 (6.4075, 7.4725)
  point P6 (21.8975, 7.4725)
  point P7 (6.4075, -16.0275)
  point P8 (21.8975, -16.0275)
  point P9 (33.3275, 11.9525)
  point P10 (33.3275, 0.5225)
  point P11 (33.3275, -10.9075)
  point P12 (30.8275, -23.6475)
  dimension "d14" = 3
  dimension "d15" = 3
  dimension "d16" = 2
  dimension "d17" = 2
  dimension "d18" = 2
  dimension "d19" = 2
  dimension "d20" = 2
  dimension "d21" = 2
  dimension "d22" = 4
  dimension "d23" = 4
  dimension "d24" = 4
  dimension "d25" = 4
  constraints: 96 end point, 48 point on circle, 48 tangent, 24 centre point, 21 parallel, 12 midpoint, 2 vertical, 1 perpendicular
  measures "d14" diameter of A107
  measures "d15" diameter of A109
  measures "d16" diameter of A111
  measures "d17" diameter of A113
  measures "d18" diameter of A115
  measures "d19" diameter of A117
  measures "d20" diameter of A119
  measures "d21" diameter of A121
  measures "d22" diameter of A123
  measures "d23" diameter of A125
  measures "d24" diameter of A127
  measures "d25" diameter of A129
extrude "Extrusion5" cut sketch "Sketch5" against normal blind 14 contours A6 | A7 | A8 | A9 | A10 | A11 | A12 | A13 | A14 | A15 | A16 | A17 | A18 | A19 | A20 | A21 | A22 | A23 | A24 | A25 | A26 | A27 | A28 | A29 | A30 | A31 | A32 | A33 | A34 | A35 | A36 | A37 | A38 | A39 | A40 | A41 | A42 | A43 | A44 | A45 | A46 | A47 | A48 | A49 | A50 | A51 | A52 | A53 | A54 | A55 | A56 | A57 | A58 | A59 | A60 | A61 | A62 | A63 | A64 | A65 | A66 | A67 | A68 | A69 | A70 | A71 | A72 | A73 | A74 | A75 | A76 | A77 | A78 | A79 | A80 | A81 | A82 | A83 | A84 | A85 | A86 | A87 | A88 | A89 | A90 | A91 | A92 | A93 | A94 | A95 | A96 | A97 | A98 | A99 | A106 L6 A107 L5 | A108 L9 A109 L8 | A110 L12 A111 L11 | A112 L15 A113 L14 | A114 L18 A115 L17 | A116 L21 A117 L20 | A118 L24 A119 L23 | A120 L27 A121 L26 | A122 L30 A123 L29 | A124 L33 A125 L32 | A126 L36 A127 L35 | A128 L39 A129 L38
sketch "Sketch6" plane through (0, 0, 3) normal (0, 0, 1) x (1, 0, 0)
  arc A0 (-14.0225, -21.7475) -> (-12.0225, -21.7475) centre (-13.0225, -21.7475) ccw projected
  line L0 (-14.0225, -21.7475) -> (-14.0225, 13.8125) projected
  arc A1 (-12.0225, 13.8125) -> (-14.0225, 13.8125) centre (-13.0225, 13.8125) ccw projected
  line L1 (-12.0225, 13.8125) -> (-12.0225, -21.7475) projected
  line L2 (22.8975, 16.3625) -> (22.8975, -1.4175) projected
  arc A2 (20.8975, -1.4175) -> (22.8975, -1.4175) centre (21.8975, -1.4175) ccw projected
  line L3 (20.8975, -1.4175) -> (20.8975, 16.3625) projected
  arc A3 (22.8975, 16.3625) -> (20.8975, 16.3625) centre (21.8975, 16.3625) ccw projected
  line L4 (31.3275, -13.4075) -> (31.3275, -8.4075) projected
  arc A4 (35.3275, -8.4075) -> (31.3275, -8.4075) centre (33.3275, -8.4075) ccw projected
  line L5 (35.3275, -8.4075) -> (35.3275, -13.4075) projected
  arc A5 (31.3275, -13.4075) -> (35.3275, -13.4075) centre (33.3275, -13.4075) ccw projected
  line L6 (31.3275, -1.9775) -> (31.3275, 3.0225) projected
  arc A6 (35.3275, 3.0225) -> (31.3275, 3.0225) centre (33.3275, 3.0225) ccw projected
  line L7 (35.3275, 3.0225) -> (35.3275, -1.9775) projected
  arc A7 (31.3275, -1.9775) -> (35.3275, -1.9775) centre (33.3275, -1.9775) ccw projected
  arc A8 (5.4075, -24.9175) -> (7.4075, -24.9175) centre (6.4075, -24.9175) ccw projected
  line L8 (5.4075, -24.9175) -> (5.4075, -7.1375) projected
  arc A9 (7.4075, -7.1375) -> (5.4075, -7.1375) centre (6.4075, -7.1375) ccw projected
  line L9 (7.4075, -7.1375) -> (7.4075, -24.9175) projected
  arc A10 (-19.6125, -17.2975) -> (-16.6125, -17.2975) centre (-18.1125, -17.2975) ccw projected
  line L10 (-19.6125, -17.2975) -> (-19.6125, 10.6425) projected
  arc A11 (-16.6125, 10.6425) -> (-19.6125, 10.6425) centre (-18.1125, 10.6425) ccw projected
  line L11 (-16.6125, 10.6425) -> (-16.6125, -17.2975) projected
  line L12 (1.2075, -21.7475) -> (1.2075, 13.8125) projected
  arc A12 (3.2075, 13.8125) -> (1.2075, 13.8125) centre (2.2075, 13.8125) ccw projected
  line L13 (3.2075, 13.8125) -> (3.2075, -21.7475) projected
  arc A13 (1.2075, -21.7475) -> (3.2075, -21.7475) centre (2.2075, -21.7475) ccw projected
  arc A14 (22.8975, -7.1375) -> (20.8975, -7.1375) centre (21.8975, -7.1375) ccw projected
  line L14 (22.8975, -7.1375) -> (22.8975, -24.9175) projected
  arc A15 (20.8975, -24.9175) -> (22.8975, -24.9175) centre (21.8975, -24.9175) ccw projected
  line L15 (20.8975, -24.9175) -> (20.8975, -7.1375) projected
  arc A16 (28.3275, -21.6475) -> (28.3275, -25.6475) centre (28.3275, -23.6475) ccw projected
  line L16 (28.3275, -21.6475) -> (33.3275, -21.6475) projected
  arc A17 (33.3275, -25.6475) -> (33.3275, -21.6475) centre (33.3275, -23.6475) ccw projected
  line L17 (33.3275, -25.6475) -> (28.3275, -25.6475) projected
  arc A18 (35.3275, 14.4525) -> (31.3275, 14.4525) centre (33.3275, 14.4525) ccw projected
  line L18 (35.3275, 14.4525) -> (35.3275, 9.4525) projected
  arc A19 (31.3275, 9.4525) -> (35.3275, 9.4525) centre (33.3275, 9.4525) ccw projected
  line L19 (31.3275, 9.4525) -> (31.3275, 14.4525) projected
  line L20 (7.4075, 16.3625) -> (7.4075, -1.4175) projected
  arc A20 (5.4075, -1.4175) -> (7.4075, -1.4175) centre (6.4075, -1.4175) ccw projected
  line L21 (5.4075, -1.4175) -> (5.4075, 16.3625) projected
  arc A21 (7.4075, 16.3625) -> (5.4075, 16.3625) centre (6.4075, 16.3625) ccw projected
  line L22 (-31.8425, 10.6425) -> (-31.8425, -17.2975) projected
  arc A22 (-34.8425, -17.2975) -> (-31.8425, -17.2975) centre (-33.3425, -17.2975) ccw projected
  line L23 (-34.8425, -17.2975) -> (-34.8425, 10.6425) projected
  arc A23 (-31.8425, 10.6425) -> (-34.8425, 10.6425) centre (-33.3425, 10.6425) ccw projected
  circle A24 centre (-25.7325, -16.0275) radius 1.27 projected
  circle A25 centre (-25.7325, 9.3725) radius 1.27 projected
  circle A26 centre (-13.0275, -24.2825) radius 0.889 projected
  circle A27 centre (2.2125, 16.3575) radius 0.889 projected
  circle A28 centre (2.2125, -24.2825) radius 0.889 projected
  circle A29 centre (-13.0275, 16.3575) radius 0.889 projected
  line L24 (-42, -31.5) -> (42, -31.5) projected
  line L25 (42, -31.5) -> (42, 31.5) projected
  line L26 (42, 31.5) -> (-42, 31.5) projected
  line L27 (-42, 31.5) -> (-42, -31.5) projected
  circle A30 centre (-13.0275, 16.3575) radius 0.889 projected
  circle A31 centre (2.2125, -24.2825) radius 0.889 projected
  line L28 (-13.0275, 16.3575) -> (2.2125, -24.2825)
  line L29 (2.2125, -24.2825) -> (2.2125, 16.3575)
  circle A32 centre (2.2125, 16.3575) radius 0.889 projected
  circle A33 centre (-13.0275, -24.2825) radius 0.889 projected
  line L30 (2.2125, 16.3575) -> (-13.0275, -24.2825)
  circle A34 centre (-5.4075, -3.9625) radius 4
  circle A35 centre (-5.4075, -13.9625) radius 4
  circle A36 centre (-5.4075, -23.9625) radius 4
  circle A37 centre (-5.4075, 6.0375) radius 4
  circle A38 centre (-5.4075, -3.9625) radius 4
  circle A39 centre (-5.4075, -13.9625) radius 4
  circle A40 centre (-5.4075, 16.0375) radius 4
  circle A41 centre (-5.4075, 6.0375) radius 4
  circle A42 centre (-5.4075, -3.9625) radius 4
  circle A43 centre (14.0925, 16.0375) radius 4
  circle A44 centre (14.0925, 6.0375) radius 4
  circle A45 centre (14.0925, -3.9625) radius 4
  circle A46 centre (14.0925, -13.9625) radius 4
  circle A47 centre (14.0925, -23.9625) radius 4
  circle A48 centre (-25.4075, 16.0375) radius 4
  circle A49 centre (-25.4075, -3.9625) radius 4
  circle A50 centre (-25.4075, -23.9625) radius 4
  point P0 (0, 0)
  dimension "d28" = 8
  dimension "d31" = 10
  dimension "d34" = 10
  dimension "d39" = 19.5
  dimension "d46" = 20
  constraints: 17 centre point, 6 end point, 3 vertical, 2 horizontal, 2 midpoint, 32 other
  measures "d28" diameter of A34
  measures "d31" distance of A34.centre A35.centre
  measures "d34" distance of A34.centre A37.centre
  measures "d39" distance of A40.centre A43.centre
  measures "d46" distance of A40.centre A48.centre
extrude "Extrusion6" cut sketch "Sketch6" against normal blind 14 contours A35 L30 | L30 A35 L28 | A37 L30 L28 | L28 A37 | L28 A35 | A37 L30 | A34 L28 L30 | L30 L28 A34 | A34 L30 L28 | L30 A34 L28 | A36 | A40 | A43 | A44 | A45 | A46 | A47 | A48 | A49 | A50
sketch "Sketch7" plane through (0, 0, 3) normal (0, 0, 1) x (1, 0, 0)
  circle A0 centre (-25.4075, -23.9625) radius 4 projected
  circle A1 centre (-5.4075, -13.9625) radius 4 projected
  circle A2 centre (14.0925, -3.9625) radius 4 projected
  circle A3 centre (14.0925, 6.0375) radius 4 projected
  circle A4 centre (-5.4075, -23.9625) radius 4 projected
  circle A5 centre (-5.4075, 16.0375) radius 4 projected
  circle A6 centre (-25.4075, -3.9625) radius 4 projected
  circle A7 centre (-5.4075, -3.9625) radius 4 projected
  circle A8 centre (14.0925, -13.9625) radius 4 projected
  circle A9 centre (14.0925, 16.0375) radius 4 projected
  circle A10 centre (14.0925, -23.9625) radius 4 projected
  circle A11 centre (-5.4075, 6.0375) radius 4 projected
  circle A12 centre (-25.4075, 16.0375) radius 4 projected
  arc A13 (-14.0225, -21.7475) -> (-12.0225, -21.7475) centre (-13.0225, -21.7475) ccw projected
  line L0 (-14.0225, -21.7475) -> (-14.0225, 13.8125) projected
  arc A14 (-12.0225, 13.8125) -> (-14.0225, 13.8125) centre (-13.0225, 13.8125) ccw projected
  line L1 (-12.0225, 13.8125) -> (-12.0225, -21.7475) projected
  line L2 (22.8975, 16.3625) -> (22.8975, -1.4175) projected
  arc A15 (20.8975, -1.4175) -> (22.8975, -1.4175) centre (21.8975, -1.4175) ccw projected
  line L3 (20.8975, -1.4175) -> (20.8975, 16.3625) projected
  arc A16 (22.8975, 16.3625) -> (20.8975, 16.3625) centre (21.8975, 16.3625) ccw projected
  line L4 (31.3275, -13.4075) -> (31.3275, -8.4075) projected
  arc A17 (35.3275, -8.4075) -> (31.3275, -8.4075) centre (33.3275, -8.4075) ccw projected
  line L5 (35.3275, -8.4075) -> (35.3275, -13.4075) projected
  arc A18 (31.3275, -13.4075) -> (35.3275, -13.4075) centre (33.3275, -13.4075) ccw projected
  line L6 (31.3275, -1.9775) -> (31.3275, 3.0225) projected
  arc A19 (35.3275, 3.0225) -> (31.3275, 3.0225) centre (33.3275, 3.0225) ccw projected
  line L7 (35.3275, 3.0225) -> (35.3275, -1.9775) projected
  arc A20 (31.3275, -1.9775) -> (35.3275, -1.9775) centre (33.3275, -1.9775) ccw projected
  arc A21 (5.4075, -24.9175) -> (7.4075, -24.9175) centre (6.4075, -24.9175) ccw projected
  line L8 (5.4075, -24.9175) -> (5.4075, -7.1375) projected
  arc A22 (7.4075, -7.1375) -> (5.4075, -7.1375) centre (6.4075, -7.1375) ccw projected
  line L9 (7.4075, -7.1375) -> (7.4075, -24.9175) projected
  arc A23 (-19.6125, -17.2975) -> (-16.6125, -17.2975) centre (-18.1125, -17.2975) ccw projected
  line L10 (-19.6125, -17.2975) -> (-19.6125, 10.6425) projected
  arc A24 (-16.6125, 10.6425) -> (-19.6125, 10.6425) centre (-18.1125, 10.6425) ccw projected
  line L11 (-16.6125, 10.6425) -> (-16.6125, -17.2975) projected
  line L12 (1.2075, -21.7475) -> (1.2075, 13.8125) projected
  arc A25 (3.2075, 13.8125) -> (1.2075, 13.8125) centre (2.2075, 13.8125) ccw projected
  line L13 (3.2075, 13.8125) -> (3.2075, -21.7475) projected
  arc A26 (1.2075, -21.7475) -> (3.2075, -21.7475) centre (2.2075, -21.7475) ccw projected
  arc A27 (22.8975, -7.1375) -> (20.8975, -7.1375) centre (21.8975, -7.1375) ccw projected
  line L14 (22.8975, -7.1375) -> (22.8975, -24.9175) projected
  arc A28 (20.8975, -24.9175) -> (22.8975, -24.9175) centre (21.8975, -24.9175) ccw projected
  line L15 (20.8975, -24.9175) -> (20.8975, -7.1375) projected
  arc A29 (28.3275, -21.6475) -> (28.3275, -25.6475) centre (28.3275, -23.6475) ccw projected
  line L16 (28.3275, -21.6475) -> (33.3275, -21.6475) projected
  arc A30 (33.3275, -25.6475) -> (33.3275, -21.6475) centre (33.3275, -23.6475) ccw projected
  line L17 (33.3275, -25.6475) -> (28.3275, -25.6475) projected
  arc A31 (35.3275, 14.4525) -> (31.3275, 14.4525) centre (33.3275, 14.4525) ccw projected
  line L18 (35.3275, 14.4525) -> (35.3275, 9.4525) projected
  arc A32 (31.3275, 9.4525) -> (35.3275, 9.4525) centre (33.3275, 9.4525) ccw projected
  line L19 (31.3275, 9.4525) -> (31.3275, 14.4525) projected
  line L20 (7.4075, 16.3625) -> (7.4075, -1.4175) projected
  arc A33 (5.4075, -1.4175) -> (7.4075, -1.4175) centre (6.4075, -1.4175) ccw projected
  line L21 (5.4075, -1.4175) -> (5.4075, 16.3625) projected
  arc A34 (7.4075, 16.3625) -> (5.4075, 16.3625) centre (6.4075, 16.3625) ccw projected
  line L22 (-31.8425, 10.6425) -> (-31.8425, -17.2975) projected
  arc A35 (-34.8425, -17.2975) -> (-31.8425, -17.2975) centre (-33.3425, -17.2975) ccw projected
  line L23 (-34.8425, -17.2975) -> (-34.8425, 10.6425) projected
  arc A36 (-31.8425, 10.6425) -> (-34.8425, 10.6425) centre (-33.3425, 10.6425) ccw projected
  circle A37 centre (-25.7325, -16.0275) radius 1.27 projected
  circle A38 centre (-25.7325, 9.3725) radius 1.27 projected
  circle A39 centre (-13.0275, -24.2825) radius 0.889 projected
  circle A40 centre (2.2125, 16.3575) radius 0.889 projected
  circle A41 centre (2.2125, -24.2825) radius 0.889 projected
  circle A42 centre (-13.0275, 16.3575) radius 0.889 projected
  line L24 (-42, -31.5) -> (42, -31.5) projected
  line L25 (42, -31.5) -> (42, 31.5) projected
  line L26 (42, 31.5) -> (-42, 31.5) projected
  line L27 (-42, 31.5) -> (-42, -31.5) projected
  line L28 (-25.4075, 1.0375) -> (-25.4075, -8.9625) construction
  line L29 (-29.4075, 1.0375) -> (-29.4075, -8.9625)
  line L30 (-21.4075, -8.9625) -> (-21.4075, 1.0375)
  arc A43 (-21.4075, 1.0375) -> (-29.4075, 1.0375) centre (-25.4075, 1.0375) ccw
  arc A44 (-29.4075, -8.9625) -> (-21.4075, -8.9625) centre (-25.4075, -8.9625) ccw
  point P0 (0, 0)
  point P1 (-29.4075, -3.9625)
  point P2 (-21.4075, -3.9625)
  dimension "d53" = 5
  dimension "d54" = 8
  constraints: 8 end point, 4 point on circle, 4 tangent, 2 centre point, 1 midpoint, 1 parallel, 1 vertical
  measures "d53" distance of A6.centre L28.end
  measures "d54" diameter of A44
extrude "Extrusion7" cut sketch "Sketch7" against normal blind 14 contours L30 A44 L29 A6 | A6 L29 A43 L30
sketch "Sketch9" plane through (0, 0, 3) normal (0, 0, 1) x (1, 0, 0)
  point P0 (0, 0)
sketch "Sketch11" plane through (0, 0, 3) normal (0, 0, 1) x (1, 0, 0)
  line L0 (-21.4075, 1.0375) -> (-21.4075, -8.9625) projected
  arc A0 (-29.4075, -8.9625) -> (-21.4075, -8.9625) centre (-25.4075, -8.9625) ccw projected
  line L1 (-29.4075, -8.9625) -> (-29.4075, 1.0375) projected
  arc A1 (-21.4075, 1.0375) -> (-29.4075, 1.0375) centre (-25.4075, 1.0375) ccw projected
  circle A2 centre (-25.4075, -23.9625) radius 4 projected
  circle A3 centre (-5.4075, -13.9625) radius 4 projected
  circle A4 centre (14.0925, -3.9625) radius 4 projected
  circle A5 centre (14.0925, 6.0375) radius 4 projected
  circle A6 centre (-5.4075, -23.9625) radius 4 projected
  circle A7 centre (-5.4075, 16.0375) radius 4 projected
  circle A8 centre (-5.4075, -3.9625) radius 4 projected
  circle A9 centre (14.0925, -13.9625) radius 4 projected
  circle A10 centre (14.0925, 16.0375) radius 4 projected
  circle A11 centre (14.0925, -23.9625) radius 4 projected
  circle A12 centre (-5.4075, 6.0375) radius 4 projected
  circle A13 centre (-25.4075, 16.0375) radius 4 projected
  arc A14 (-14.0225, -21.7475) -> (-12.0225, -21.7475) centre (-13.0225, -21.7475) ccw projected
  line L2 (-14.0225, -21.7475) -> (-14.0225, 13.8125) projected
  arc A15 (-12.0225, 13.8125) -> (-14.0225, 13.8125) centre (-13.0225, 13.8125) ccw projected
  line L3 (-12.0225, 13.8125) -> (-12.0225, -21.7475) projected
  line L4 (22.8975, 16.3625) -> (22.8975, -1.4175) projected
  arc A16 (20.8975, -1.4175) -> (22.8975, -1.4175) centre (21.8975, -1.4175) ccw projected
  line L5 (20.8975, -1.4175) -> (20.8975, 16.3625) projected
  arc A17 (22.8975, 16.3625) -> (20.8975, 16.3625) centre (21.8975, 16.3625) ccw projected
  line L6 (31.3275, -13.4075) -> (31.3275, -8.4075) projected
  arc A18 (35.3275, -8.4075) -> (31.3275, -8.4075) centre (33.3275, -8.4075) ccw projected
  line L7 (35.3275, -8.4075) -> (35.3275, -13.4075) projected
  arc A19 (31.3275, -13.4075) -> (35.3275, -13.4075) centre (33.3275, -13.4075) ccw projected
  line L8 (31.3275, -1.9775) -> (31.3275, 3.0225) projected
  arc A20 (35.3275, 3.0225) -> (31.3275, 3.0225) centre (33.3275, 3.0225) ccw projected
  line L9 (35.3275, 3.0225) -> (35.3275, -1.9775) projected
  arc A21 (31.3275, -1.9775) -> (35.3275, -1.9775) centre (33.3275, -1.9775) ccw projected
  arc A22 (5.4075, -24.9175) -> (7.4075, -24.9175) centre (6.4075, -24.9175) ccw projected
  line L10 (5.4075, -24.9175) -> (5.4075, -7.1375) projected
  arc A23 (7.4075, -7.1375) -> (5.4075, -7.1375) centre (6.4075, -7.1375) ccw projected
  line L11 (7.4075, -7.1375) -> (7.4075, -24.9175) projected
  arc A24 (-19.6125, -17.2975) -> (-16.6125, -17.2975) centre (-18.1125, -17.2975) ccw projected
  line L12 (-19.6125, -17.2975) -> (-19.6125, 10.6425) projected
  arc A25 (-16.6125, 10.6425) -> (-19.6125, 10.6425) centre (-18.1125, 10.6425) ccw projected
  line L13 (-16.6125, 10.6425) -> (-16.6125, -17.2975) projected
  line L14 (1.2075, -21.7475) -> (1.2075, 13.8125) projected
  arc A26 (3.2075, 13.8125) -> (1.2075, 13.8125) centre (2.2075, 13.8125) ccw projected
  line L15 (3.2075, 13.8125) -> (3.2075, -21.7475) projected
  arc A27 (1.2075, -21.7475) -> (3.2075, -21.7475) centre (2.2075, -21.7475) ccw projected
  arc A28 (22.8975, -7.1375) -> (20.8975, -7.1375) centre (21.8975, -7.1375) ccw projected
  line L16 (22.8975, -7.1375) -> (22.8975, -24.9175) projected
  arc A29 (20.8975, -24.9175) -> (22.8975, -24.9175) centre (21.8975, -24.9175) ccw projected
  line L17 (20.8975, -24.9175) -> (20.8975, -7.1375) projected
  arc A30 (28.3275, -21.6475) -> (28.3275, -25.6475) centre (28.3275, -23.6475) ccw projected
  line L18 (28.3275, -21.6475) -> (33.3275, -21.6475) projected
  arc A31 (33.3275, -25.6475) -> (33.3275, -21.6475) centre (33.3275, -23.6475) ccw projected
  line L19 (33.3275, -25.6475) -> (28.3275, -25.6475) projected
  arc A32 (35.3275, 14.4525) -> (31.3275, 14.4525) centre (33.3275, 14.4525) ccw projected
  line L20 (35.3275, 14.4525) -> (35.3275, 9.4525) projected
  arc A33 (31.3275, 9.4525) -> (35.3275, 9.4525) centre (33.3275, 9.4525) ccw projected
  line L21 (31.3275, 9.4525) -> (31.3275, 14.4525) projected
  line L22 (7.4075, 16.3625) -> (7.4075, -1.4175) projected
  arc A34 (5.4075, -1.4175) -> (7.4075, -1.4175) centre (6.4075, -1.4175) ccw projected
  line L23 (5.4075, -1.4175) -> (5.4075, 16.3625) projected
  arc A35 (7.4075, 16.3625) -> (5.4075, 16.3625) centre (6.4075, 16.3625) ccw projected
  line L24 (-31.8425, 10.6425) -> (-31.8425, -17.2975) projected
  arc A36 (-34.8425, -17.2975) -> (-31.8425, -17.2975) centre (-33.3425, -17.2975) ccw projected
  line L25 (-34.8425, -17.2975) -> (-34.8425, 10.6425) projected
  arc A37 (-31.8425, 10.6425) -> (-34.8425, 10.6425) centre (-33.3425, 10.6425) ccw projected
  circle A38 centre (-25.7325, -16.0275) radius 1.27 projected
  circle A39 centre (-25.7325, 9.3725) radius 1.27 projected
  circle A40 centre (-13.0275, -24.2825) radius 0.889 projected
  circle A41 centre (2.2125, 16.3575) radius 0.889 projected
  circle A42 centre (2.2125, -24.2825) radius 0.889 projected
  circle A43 centre (-13.0275, 16.3575) radius 0.889 projected
  line L26 (-42, -31.5) -> (42, -31.5) projected
  line L27 (42, -31.5) -> (42, 31.5) projected
  line L28 (42, 31.5) -> (-42, 31.5) projected
  line L29 (-42, 31.5) -> (-42, -31.5) projected
  line L30 (42, 31.5) -> (42, -31.5) projected
  line L31 (42, -31.5) -> (32, -31.5)
  line L32 (-42, -31.5) -> (42, -31.5) projected
  line L33 (42, -31.5) -> (42, -21.5)
  line L34 (42, -21.5) -> (32, -31.5)
  line L35 (-42, 31.5) -> (-42, -31.5) projected
  line L36 (-42, -31.5) -> (-32, -31.5)
  line L37 (-42, -31.5) -> (-42, -21.5)
  line L38 (42, 31.5) -> (-42, 31.5) projected
  line L39 (42, 31.5) -> (42, 21.5)
  line L40 (42, 31.5) -> (32, 31.5)
  line L41 (-42, 31.5) -> (-42, 21.5)
  line L42 (-42, 31.5) -> (-32, 31.5)
  line L43 (-32, -31.5) -> (-42, -21.5)
  line L44 (-42, 21.5) -> (-32, 31.5)
  line L45 (42, 21.5) -> (32, 31.5)
  point P0 (0, 0)
  dimension "d74" = 10
  dimension "d75" = 10
  dimension "d76" = 10
  dimension "d77" = 10
  dimension "d78" = 10
  dimension "d79" = 10
  dimension "d80" = 10
  dimension "d81" = 10
  constraints: 24 end point, 8 point on line
  measures "d74" distance of L26.end L31.end
  measures "d75" distance of L26.end L33.end
  measures "d76" distance of L26.start L36.end
  measures "d77" distance of L26.start L37.end
  measures "d78" distance of L27.end L39.end
  measures "d79" distance of L27.end L40.end
  measures "d80" distance of L28.end L41.end
  measures "d81" distance of L28.end L42.end
extrude "Extrusion10" cut sketch "Sketch11" against normal blind 20 contours L29 L43 L26 | L34 L27 L26 | L29 L28 L44 | L45 L28 L27
chamfer "Chamfer1" distance 0.5 angle 45 48 edges at (33.3275, 7.4525, 0) (35.3275, 11.9525, 0) (33.3275, 16.4525, 0) (31.3275, 11.9525, 0) (33.3275, 5.0225, 0) (31.3275, 0.5225, 0) (33.3275, -3.9775, 0) (35.3275, 0.5225, 0) (33.3275, -6.4075, 0) (31.3275, -10.9075, 0) (33.3275, -15.4075, 0) (35.3275, -10.9075, 0) (30.8275, -21.6475, 0) (26.3275, -23.6475, 0) (30.8275, -25.6475, 0) (35.3275, -23.6475, 0) (22.8975, -16.0275, 0) (21.8975, -6.1375, 0) (20.8975, -16.0275, 0) (21.8975, -25.9175, 0) (21.8975, -2.4175, 0) (22.8975, 7.4725, 0) (21.8975, 17.3625, 0) (20.8975, 7.4725, 0) (6.4075, -2.4175, 0) (7.4075, 7.4725, 0) (6.4075, 17.3625, 0) (5.4075, 7.4725, 0) (6.4075, -6.1375, 0) (5.4075, -16.0275, 0) (6.4075, -25.9175, 0) (7.4075, -16.0275, 0) (3.2075, -3.9675, 0) (2.2075, 14.8125, 0) (1.2075, -3.9675, 0) (2.2075, -22.7475, 0) (-12.0225, -3.9675, 0) (-13.0225, 14.8125, 0) (-14.0225, -3.9675, 0) (-13.0225, -22.7475, 0) (-16.6125, -3.3275, 0) (-18.1125, 12.1425, 0) (-19.6125, -3.3275, 0) (-18.1125, -18.7975, 0) (-31.8425, -3.3275, 0) (-33.3425, 12.1425, 0) (-34.8425, -3.3275, 0) (-33.3425, -18.7975, 0)